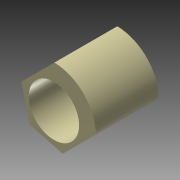
# Autodesk Inventor part: NutInserperFilling
Saved by Autodesk Inventor 2015 (Build 190159000, 159)
## iProperties
Created: 2015-04-23
Part Number: NutInserperFilling
Material: Nylon 6/6
Document SubType Name: Modeling
Designer: Akovo_000
Density: 1.13 g/cm^3
Appearance: Nylon 6
Mass: 0.0623402 g
Surface Area: 1.74965 cm^2
Volume: 0.0551683 cm^3
Author: Akovo_000
Autodesk Inventor part; units mm, degrees
ref_plane "YZ Plane" through (0, 0, 0) normal (1, 0, 0) x (0, 1, 0)
ref_plane "XZ Plane" through (0, 0, 0) normal (0, 1, 0) x (-1, 0, 0)
ref_plane "XY Plane" through (0, 0, 0) normal (0, 0, 1) x (1, 0, 0)
sketch "Sketch1" plane through (0, 0, 0) normal (0, 1, 0) x (-1, 0, 0)
  arc A0 (-7.3333, 0) -> (-10.6667, -3.3333) centre (-7.3333, -3.3333) ccw
  arc A1 (-7.3333, 0) -> (-7.3667, -0.0002) centre (-7.3333, -3.3333) ccw
  line L0 (-5.4282, -5.2385) -> (-8.0307, -5.9358)
  line L1 (-8.0307, -5.9358) -> (-5.4282, -5.2385)
  line L2 (-8.0307, -5.9358) -> (-9.9358, -4.0307)
  line L3 (-6.636, -0.7308) -> (-4.7308, -2.636)
  line L4 (-4.7308, -2.636) -> (-5.4282, -5.2385)
  line L5 (-8.0307, -5.9358) -> (-9.9358, -4.0307)
  line L6 (-6.636, -0.7308) -> (-4.7308, -2.636)
  line L7 (-6.636, -0.7308) -> (-7.3667, -0.0002)
  line L8 (-9.9358, -4.0307) -> (-10.6665, -3.3)
  arc A2 (-10.6665, -3.3) -> (-10.6667, -3.3333) centre (-7.3333, -3.3333) ccw
  arc A3 (-7.3667, -0.0002) -> (-10.6665, -3.3) centre (-7.3333, -3.3333) ccw construction
  circle A4 centre (-7.3333, -3.3333) radius 2
  point P0 (0, 0)
  dimension "d2" = 4
  constraints: 18 end point, 11 point on circle, 5 centre point, 2 coincident, 2 collinear, 2 equal length
  measures "d2" diameter of A4
extrude "Extrusion1" add sketch "Sketch1" along normal blind 5
body "Solid1"
